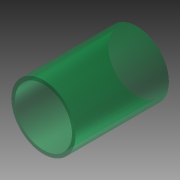
# Autodesk Inventor part: TU-004
Saved by Autodesk Inventor 2011 (Build 150229000, 229)
## iProperties
Shininess: 64.0
Angle Display Precision: 2
Document Length Units: 11269
Document Angle Units: 11279
Document Time Units: 11290
Document Mass Units: 11286
Document Length Units Precision: 3
Document Angle Units Precision: 2
Created: 2002-07-24
Part Number: TU-004
Document SubType Name: Modeling
Designer: PN
Description: Cylinder Tube
Density: 8.08 g/cm^3
Mass: 184.955 g
Surface Area: 189.956 cm^2
Volume: 22.8904 cm^3
Material: Stainless Steel
Density: 0.0
Volumn: 0.0
Area: 0.0
PropertySet Name: Model Information
Control State: 0
Master: False
Checked Out: False
LENGTH: 1.000 in
Author: PN
Autodesk Inventor part; units mm, degrees
ref_plane "YZ Plane" through (0, 0, 0) normal (1, 0, 0) x (0, 1, 0)
ref_plane "XZ Plane" through (0, 0, 0) normal (0, 1, 0) x (-1, 0, 0)
ref_plane "XY Plane" through (0, 0, 0) normal (0, 0, 1) x (1, 0, 0)
sketch "Sketch1" plane through (0, 0, 0) normal (0, 0, 1) x (1, 0, 0)
  circle A0 centre (0, 0) radius 23
  circle A1 centre (0, 0) radius 20.5
  dimension "d0" = 46
  dimension "d1" = 41
  constraints: 2 centre point, 2 coincident
  measures "d0" diameter of A0
  measures "d1" diameter of A1
extrude "Extrusion1" add sketch "Sketch1" along normal mid plane 67
equation "\"LENGTH\" = 25.4"
body "Solid1"
